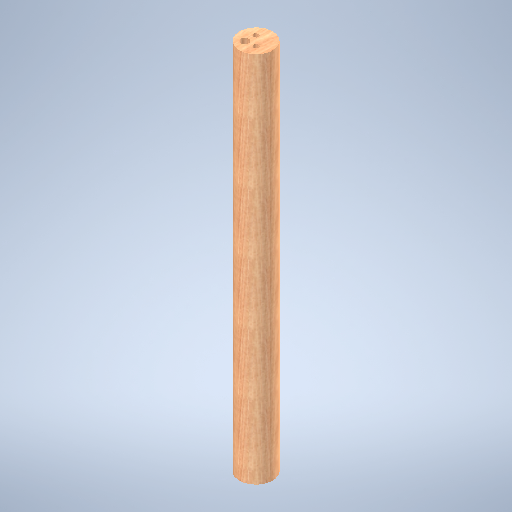
# Autodesk Inventor part: Dowel2
Saved by Autodesk Inventor 2025.3 (Build 293356000, 356)
## iProperties
Created: 2026-01-15
Part Number: Dowel2
Material: Generic
Document SubType Name: Modeling
Designer: Balint
Density: 1 g/cm^3
Appearance: Red Birch
Mass: 128.439 g
Surface Area: 293.403 cm^2
Volume: 128.439 cm^3
Author: Balint
Autodesk Inventor part; units mm, degrees
ref_plane "YZ Plane" through (0, 0, 0) normal (1, 0, 0) x (0, 1, 0)
ref_plane "XZ Plane" through (0, 0, 0) normal (0, 1, 0) x (-1, 0, 0)
ref_plane "XY Plane" through (0, 0, 0) normal (0, 0, 1) x (1, 0, 0)
sketch "Sketch1" plane through (0, 0, 0) normal (0, 1, 0) x (-1, 0, 0)
  circle A0 centre (0, 0) radius 12.5
  dimension "d0" = 25
  constraints: 1 centre point, 1 coincident
  measures "d0" diameter of A0
extrude "Extrusion1" add sketch "Sketch1" along normal blind 280
sketch "Sketch2" plane through (0, 0, 0) normal (0, -1, 0) x (1, 0, 0)
  line L0 (-3.5355, -3.5355) -> (3.5355, 3.5355)
  line L1 (-3.5355, -3.5355) -> (6.4645, -3.5355) construction
  circle A0 centre (-3.5355, -3.5355) radius 1.9
  circle A1 centre (3.5355, 3.5355) radius 1.9
  point P0 (0, 0)
  dimension "d3" = 10
  dimension "d4" = 45
  dimension "d5" = 3.8
  dimension "d6" = 3.8
  constraints: 4 end point, 2 centre point, 2 coincident, 1 equal length, 1 horizontal, 1 midpoint
  measures "d3" distance of L0.start L0.end
  measures "d4" angle of L1 L0
  measures "d5" diameter of A0
  measures "d6" diameter of A1
extrude "Extrusion2" cut sketch "Sketch2" against normal blind 40
sketch "Sketch3" plane through (0, 0, 0) normal (0, -1, 0) x (1, 0, 0)
  line L0 (0, 0) -> (-4.2426, 4.2426)
  line L1 (0, 0) -> (6, 0) construction
  circle A0 centre (-4.2426, 4.2426) radius 3
  dimension "d9" = 6
  dimension "d10" = 135
  dimension "d11" = 6
  constraints: 4 end point, 1 centre point, 1 coincident, 1 equal length, 1 horizontal
  measures "d9" distance of L0.start L0.end
  measures "d10" angle of L1 L0
  measures "d11" diameter of A0
extrude "Extrusion3" cut sketch "Sketch3" against normal through all
sketch "Sketch6" plane through (0, 280, 0) normal (0, 1, 0) x (1, 0, 0)
  circle A0 centre (-3.5355, -3.5355) radius 1.9 construction
  circle A1 centre (3.5355, 3.5355) radius 1.9 construction
  line L0 (-3.5355, 3.5355) -> (3.5355, -3.5355)
  line L1 (-3.5355, 3.5355) -> (6.4645, 3.5355) construction
  circle A2 centre (3.5355, -3.5355) radius 2
  circle A3 centre (-3.5355, 3.5355) radius 2
  point P0 (0, 0)
  dimension "d16" = 10
  dimension "d17" = 45
  dimension "d18" = 4
  dimension "d19" = 4
  constraints: 4 end point, 2 centre point, 2 coincident, 1 equal length, 1 horizontal, 1 midpoint
  measures "d16" distance of L0.start L0.end
  measures "d17" angle of L0 L1
  measures "d18" diameter of A2
  measures "d19" diameter of A3
extrude "Extrusion4" cut sketch "Sketch6" against normal blind 8
body "Solid1"
